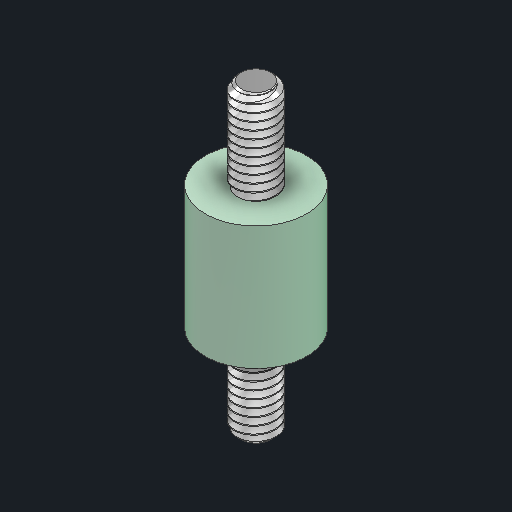
# Autodesk Inventor part: Rubber Link
Saved by Autodesk Inventor 2024 (Build 280153000, 153)
## iProperties
Created: 2021-07-20
Part Number: Rubber Link
Material: Generic
Document SubType Name: Modeling
Designer: yuany
Density: 1 g/cm^3
Appearance: Default
Author: yuany
Autodesk Inventor part; units mm, degrees
ref_plane "YZ Plane" through (0, 0, 0) normal (1, 0, 0) x (0, 1, 0)
ref_plane "XZ Plane" through (0, 0, 0) normal (0, 1, 0) x (-1, 0, 0)
ref_plane "XY Plane" through (0, 0, 0) normal (0, 0, 1) x (1, 0, 0)
sketch "Sketch1" plane through (0, 0, 0) normal (0, 1, 0) x (-1, 0, 0)
  circle A0 centre (0, 0) radius 5.207
  dimension "d0" = 10.414
  constraints: 1 centre point, 1 coincident
  measures "d0" diameter of A0
extrude "Body" add sketch "Sketch1" along normal blind 12.7
sketch "Sketch2" plane through (0, 12.7, 0) normal (0, 1, 0) x (1, 0, 0)
  circle A0 centre (0, 0) radius 1.5621
  dimension "d3" = 3.1242
  constraints: 1 centre point, 1 coincident
  measures "d3" diameter of A0
extrude "Top" add sketch "Sketch2" along normal blind 9.271
sketch "Sketch3" plane through (0, 0, 0) normal (0, -1, 0) x (1, 0, 0)
  circle A0 centre (0, 0) radius 1.5621
  dimension "d6" = 3.1242
  constraints: 1 centre point, 1 coincident
  measures "d6" diameter of A0
extrude "Bottom" add sketch "Sketch3" along normal blind 9.271
sketch "Sketch5" plane through (0, 0, 0) normal (0, 0, 1) x (1, 0, 0)
  line L0 (1.5621, 12.7) -> (1.5621, 21.971) projected
  line L1 (1.5621, 21.8948) -> (1.5621, 22.6123)
  line L2 (1.5621, 22.6123) -> (2.0955, 22.3044)
  line L3 (2.0955, 22.3044) -> (2.0955, 22.2028)
  line L4 (2.0955, 22.2028) -> (1.5621, 21.8948)
  line L5 (1.5621, 21.971) -> (-1.5621, 21.971) projected
  point P0 (0, 0)
  dimension "d21" = 60
  dimension "d22" = 0.0762
  dimension "d23" = 0.1016
  dimension "d24" = 0.5334
  constraints: 8 end point, 1 collinear, 1 equal length, 1 parallel, 1 point on line
  measures "d21" angle of L4 L2
  measures "d22" distance from line of L5 L1.start
  measures "d23" distance of L2.end L3.end
  measures "d24" distance between parallel lines of L1 L3
coil "Top Thread" sketch "Sketch5" operation add axis through (0, -10, 0) along (0, -1, 0) pitch 0.7874 turns 13.387097 hand right
sketch "Sketch4" plane through (0, 0, 0) normal (0, 0, 1) x (1, 0, 0)
  line L0 (1.5621, 0) -> (1.5621, -9.271) projected
  line L1 (1.5621, -9.1948) -> (1.5621, -9.9123)
  line L2 (1.5621, -9.9123) -> (2.0955, -9.6044)
  line L3 (2.0955, -9.6044) -> (2.0955, -9.5028)
  line L4 (2.0955, -9.5028) -> (1.5621, -9.1948)
  line L5 (-1.5621, -9.271) -> (1.5621, -9.271) projected
  point P0 (0, 0)
  dimension "d9" = 0.1016
  dimension "d10" = 60
  dimension "d11" = 0.5334
  dimension "d12" = 0.0762
  constraints: 8 end point, 1 equal length, 1 parallel, 1 point on line, 1 vertical
  measures "d9" distance of L2.end L3.end
  measures "d10" angle of L4 L2
  measures "d11" distance between parallel lines of L1 L3
  measures "d12" distance from line of L1.start L5
coil "Bottom Thread" sketch "Sketch4" operation add axis through (0, -10, 0) along (0, 1, 0) pitch 0.7874 turns 13.387097 hand right
sketch "Sketch6" plane through (0, 0, 0) normal (0, 0, 1) x (1, 0, 0)
  line L0 (0, -9.271) -> (1.4986, -9.271)
  line L1 (1.4986, -9.271) -> (2.3254, -8.4442)
  line L2 (2.3254, -8.4442) -> (2.3254, -10.3245)
  line L3 (-1.5621, -9.271) -> (1.5621, -9.271) projected
  line L4 (2.3254, -10.3245) -> (1.2681, -10.3245)
  line L5 (1.2681, -10.3245) -> (1.5621, -9.271)
  line L6 (0, -16.9119) -> (0, 29.1997) projected
  line L7 (1.5621, 21.971) -> (-1.5621, 21.971) projected
  line L8 (0, 21.971) -> (1.5621, 21.971)
  line L9 (0, 21.971) -> (1.4986, 21.971)
  line L10 (1.4986, 21.971) -> (2.2661, 21.2035)
  line L11 (2.2661, 21.2035) -> (2.2661, 22.943)
  line L12 (2.2661, 22.943) -> (1.4986, 22.943)
  line L13 (1.4986, 22.943) -> (1.4986, 21.971)
  point P0 (0, 0)
  point P1 (0.6156, -9.271)
  point P2 (0.6156, 21.971)
  dimension "d33" = 1.4986
  dimension "d34" = 135
  dimension "d35" = 0
  dimension "d36" = 0
  dimension "d38" = 1.4986
  dimension "d39" = 135
  dimension "d40" = 0
  constraints: 22 end point, 4 perpendicular, 3 horizontal, 1 collinear, 1 midpoint, 1 point on line
  measures "d33" distance of L0.start L0.end
  measures "d34" angle of L0 L1
  measures "d35" horizontal distance of point (0, 0) L0.start
  measures "d36" distance between parallel lines of L3 L0
  measures "d38" distance of L9.start L9.end
  measures "d39" angle of L9 L10
  measures "d40" distance between parallel lines of L8 L9
revolve "Taper Ends" cut sketch "Sketch6" angle 360 about axis through (0, -10, 0) along (0, 1, 0)
body "Solid1"
